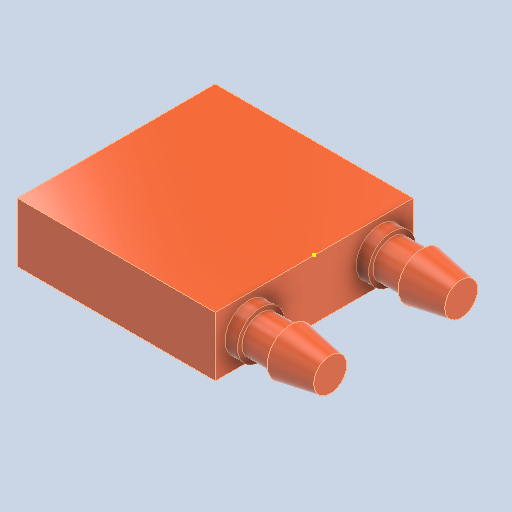
# Autodesk Inventor part: blokwodny
Saved by Autodesk Inventor 2022 (Build 260153000, 153)
## iProperties
Created: 2022-05-18
Part Number: blokwodny
Material: Żywica fenolowa
Document SubType Name: Modeling
Designer: kosak
Density: 1.38 g/cm^3
Appearance: Gładki — jasnopomarańczowy
Author: kosak
Autodesk Inventor part; units mm, degrees
ref_plane "YZ Plane" through (0, 0, 0) normal (1, 0, 0) x (0, 1, 0)
ref_plane "XZ Plane" through (0, 0, 0) normal (0, 1, 0) x (-1, 0, 0)
ref_plane "XY Plane" through (0, 0, 0) normal (0, 0, 1) x (1, 0, 0)
sketch "Szkic1" plane through (0, 0, 0) normal (0, 1, 0) x (-1, 0, 0)
  line L0 (0, 0) -> (40, 0)
  line L1 (40, 0) -> (40, 20)
  line L2 (40, 20) -> (0, 20)
  line L3 (0, 20) -> (0, 0)
  dimension "d0" = 40
  dimension "d1" = 20
  constraints: 8 end point, 2 parallel, 1 horizontal, 1 perpendicular
  measures "d0" distance of L2.end L1.end
  measures "d1" distance of L1.end L0.end
extrude "Wyciągnięcie proste1" add sketch "Szkic1" along normal blind 12
sketch "Szkic2" plane through (0, 12, 0) normal (0, 1, 0) x (1, 0, 0)
  point P0 (0, 0)
sketch "Szkic3" plane through (0, 0, 20) normal (1, 0, 0) x (0, 0, -1)
  line L0 (0, 0) -> (0, 12) projected
  line L1 (0, 6) -> (6.75, 6)
  circle A0 centre (6.75, 6) radius 4.75
  point P0 (20, 0)
  dimension "d4" = 6.75
  dimension "d5" = 9.5
  constraints: 2 end point, 1 centre point, 1 coincident, 1 horizontal, 1 midpoint
  measures "d4" distance of L1.start L1.end
  measures "d5" diameter of A0
extrude "Wyciągnięcie proste2" add sketch "Szkic3" along normal blind 2.5
sketch "Szkic4" plane through (2.5, 6, 13.25) normal (1, 0, 0) x (0, 0, -1)
  circle A0 centre (0, 0) radius 3.85
  point P0 (13.25, -6)
  dimension "d8" = 7.7
  constraints: 1 centre point
  measures "d8" diameter of A0
extrude "Wyciągnięcie proste3" add sketch "Szkic4" along normal blind 6
sketch "Szkic5" plane through (8.5, 6, 13.25) normal (1, 0, 0) x (0, 0, -1)
  circle A0 centre (0, 0) radius 4.75
  point P0 (13.25, -6)
  constraints: 1 centre point
extrude "Wyciągnięcie proste4" add sketch "Szkic5" along normal blind 8 draft -10
mirror "Odbij1" about plane through (0, 0, 0) normal (0, 0, 1) of "Wyciągnięcie proste4", "Wyciągnięcie proste3", "Wyciągnięcie proste2", "Wyciągnięcie proste1"
